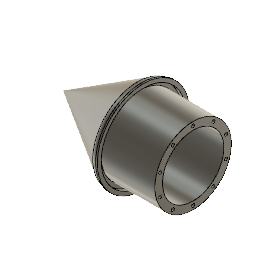
nose_cone_eng_model (Autodesk Fusion 360 design; units mm, degrees)
Autodesk Fusion 360 part; units mm, degrees
sketch "Sketch1" plane through (0, 0, 0) normal (0, 1, 0) x (1, 0, 0)
  line L0 (0.0544, -50) -> (-64.9456, -50)
  line L1 (0, -40) -> (-80, -40)
  line L2 (-64.9456, -55) -> (-64.9456, -60)
  line L3 (-64.9456, -60) -> (-67.177, -60)
  line L4 (0, 0) -> (-288.9752, 0) construction
  line L5 (0, 0) -> (187.3459, 0) construction
  line L6 (-72.3199, -58.5762) -> (-170, 0)
  arc A0 (-72.3199, -58.5762) -> (-67.177, -60) centre (-67.177, -50) ccw
  line L7 (-80, -40) -> (-80, -42.3104)
  line L8 (-80, -42.3104) -> (-150.5557, 0)
  line L9 (0, -40) -> (0.0544, -50)
  line L10 (-170, 0) -> (-150.5557, 0)
  line L11 (-64.9456, -50) -> (-69.9456, -50)
  line L12 (-69.9456, -50) -> (-69.9456, -55)
  line L13 (-69.9456, -55) -> (-64.9456, -55)
  point P0 (-69.9456, -60)
  dimension "d1" = 50
  dimension "d2" = 65
  dimension "d3" = 10
  dimension "d4" = 10
  dimension "d5" = 5
  dimension "d6" = 170
  dimension "d7" = 149.05
  dimension "d8" = 10
  dimension "d9" = 10
  dimension "d10" = 2.3104
  dimension "d11" = 5
  dimension "d12" = 5
  dimension "d13" = 5
  constraint horizontal L0
  constraint perpendicular L0 L2
  constraint perpendicular L2 L3
  constraint coincident L4.start L5.start
  constraint horizontal L4
  constraint parallel L4 L5
  constraint coincident L4 L6.end
  constraint coincident P0 L6
  constraint coincident P0 L3
  constraint tangent L6 A0
  constraint tangent L3 A0
  constraint perpendicular L1 L7
  constraint coincident L4 L8.end
  constraint parallel L6 L8
  constraint perpendicular L2 L11
  constraint perpendicular L11 L12
  constraint perpendicular L12 L13
  measures "d1" distance of L4.start L0
  measures "d2" distance of L0.start L0.end
  measures "d4" distance of L0.end L2.end
  measures "d5" distance of L2.end P0
  measures "d6" distance of L4.start L6.end
  measures "d7" angle of L4 L6
  measures "d8" radius of A0
  measures "d9" distance of L6 L8
  measures "d10" distance of L1.end L7.end
  measures "d11" distance of L12.end L2.start
  measures "d12" distance of L11.end L12.end
  measures "d13" distance of L2.end L2.start
revolve "Revolve1" add sketch "Sketch1" angle 360 about axis through (0, 0, 0) along (-1, 0, 0)
sketch "Sketch2" plane through (0, 0, 0) normal (1, 0, 0) x (0, 1, 0)
  line L0 (0, 0) -> (0, 125.4957) construction
  circle A0 centre (0, 45) radius 2
  circle A1 centre (0, 0) radius 40
  circle A2 centre (0, 0) radius 50
  circle A3 centre (0, 0) radius 40
  point P0 (0, 40)
  dimension "d15" = 4
  dimension "d16" = 5
  constraint coincident L0.start A1.centre
  constraint vertical L0
  constraint coincident L0 A0.centre
  constraint coincident L0 P0
  constraint coincident A1 P0
  measures "d15" diameter of A0
  measures "d16" distance of A0.centre P0
extrude "Extrude1" cut sketch "Sketch2" along normal mid plane 40 contours A0
pattern_circular "C-Pattern1" count 10 over 360 about axis through (1.75, 0, 0) along (1, 0, 0) of "Extrude1"
